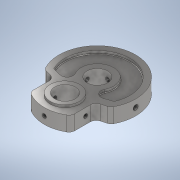
# Autodesk Inventor part: Peça10
Saved by Autodesk Inventor 2021 (Build 250183000, 183)
## iProperties
Created: 2021-07-17
Part Number: Peça10
Material: Liga de aço
Document SubType Name: Modeling
Designer: Giovanni
Density: 7.73 g/cm^3
Appearance: Semipolido
Author: Giovanni
Autodesk Inventor part; units mm, degrees
ref_plane "XZ Plane" through (0, 0, 0) normal (0, 1, 0) x (-1, 0, 0)
ref_plane "XY Plane" through (0, 0, 0) normal (0, 0, 1) x (1, 0, 0)
sketch "Esboço1" plane through (0, 0, 0) normal (0, 1, 0) x (-1, 0, 0)
  arc A0 (-55.5003, 33.8337) -> (55.5003, 33.8337) centre (0, 0) ccw
  line L0 (35, 78.734) -> (35, 47)
  line L1 (42.4118, 37.3407) -> (55.5003, 33.8337)
  line L2 (0, 0) -> (0, 90)
  arc A1 (35, 47) -> (42.4118, 37.3407) centre (45, 47) ccw
  line L3 (-35, 80.2574) -> (-35, 47)
  line L4 (-42.4118, 37.3407) -> (-55.5003, 33.8337)
  arc A2 (-42.4118, 37.3407) -> (-35, 47) centre (-45, 47) ccw
  line L5 (-35, 78.734) -> (-35, 80.2574)
  arc A3 (35, 78.734) -> (-35, 78.734) centre (0, 30) ccw
  circle A4 centre (0, 0) radius 17.5
  circle A5 centre (0, 55) radius 17.5
  point P0 (-35, 78.734)
  dimension "d6" = 65
  dimension "d7" = 90
  dimension "d8" = 35
  dimension "d9" = 105
  dimension "d10" = 10
  dimension "d11" = 47
  dimension "d12" = 10
  dimension "d13" = 35
  dimension "d14" = 105
  dimension "d15" = 60
  dimension "d16" = 35
  dimension "d17" = 55
  constraints: 12 end point, 8 point on circle, 6 centre point, 4 tangent, 4 vertical, 2 horizontal alignment, 1 coincident, 1 equal radius, 1 point on line, 1 other
  measures "d6" radius of A0
  measures "d7" distance of L2.start L2.end
  measures "d8" distance from line of L0.start L2
  measures "d9" angle of L1 L0
  measures "d10" radius of A1
  measures "d11" vertical distance of L2.start A1.centre
  measures "d12" radius of A2
  measures "d13" distance between parallel lines of L3 L2
  measures "d14" angle of L4 L3
  measures "d15" radius of A3
  measures "d16" diameter of A4
  measures "d17" distance of A5.centre L2.start
extrude "Extrusão1" add sketch "Esboço1" along normal mid plane 25
sketch "Esboço3" plane through (0, -12.5, 0) normal (0, -1, 0) x (1, 0, 0)
  arc A0 (-49.0552, 24.8713) -> (50.4541, 21.8949) centre (0, 0) ccw
  arc A1 (-23.7089, 13.9333) -> (24.4993, 12.4914) centre (0, 0) ccw
  arc A2 (-23.7089, 13.9333) -> (-34.9185, 28.6593) centre (-32.3303, 19) ccw
  line L0 (-34.9185, 28.6593) -> (-49.0552, 24.8713)
  line L1 (-42.4118, 37.3407) -> (-55.5003, 33.8337) projected
  arc A3 (36.569, 26.521) -> (24.4993, 12.4914) centre (33.4081, 17.0337) ccw
  line L2 (36.569, 26.521) -> (50.4541, 21.8949)
  dimension "d27" = 10
  dimension "d28" = 55
  dimension "d29" = 27.5
  dimension "d30" = 19
  constraints: 8 point on circle, 4 centre point, 4 end point, 4 tangent, 2 coincident, 1 equal length, 1 equal radius, 1 parallel
  measures "d27" radius of A2
  measures "d28" radius of A0
  measures "d29" radius of A1
  measures "d30" vertical distance of point (0, 0) A2.centre
extrude "Extrusão2" cut sketch "Esboço3" against normal blind 5
mirror "Espelhamento1" about plane through (0, 0, 0) normal (0, 1, 0) of "Extrusão2"
sketch "Esboço5" plane through (0, -12.5, 0) normal (0, -1, 0) x (1, 0, 0)
  circle A0 centre (0, 0) radius 23.5
  circle A1 centre (0, 0) radius 17.5 projected
  dimension "d34" = 47
  constraints: 1 centre point, 1 coincident
  measures "d34" diameter of A0
extrude "Extrusão3" add sketch "Esboço5" along normal blind 5
sketch "Esboço6" plane through (0, 12.5, 0) normal (0, 1, 0) x (1, 0, 0)
  circle A0 centre (0, -55) radius 17.5 projected
  circle A1 centre (0, -55) radius 25
  point P0 (0, 0)
  dimension "d37" = 50
  constraints: 1 centre point, 1 coincident
  measures "d37" diameter of A1
extrude "Extrusão4" add sketch "Esboço6" along normal blind 4
sketch "Esboço7" plane through (35, -12.5, 47) normal (1, 0, 0) x (0, 0, -1)
  point P0 (47, 12.5)
  point P1 (-8, 12.5)
  dimension "d40" = 55
  constraints: 1 horizontal alignment
  measures "d40" distance of point (-8, 12.5) point (47, 12.5)
hole "Furo1" at (35, 0, 55) direction (-1, 0, 0) diameter 6.917 depth 35 tip angle 118 thread size "M8x1" class "6H" standard "ANSI Metric M Profile"
pattern_circular "Padrão circular1" count 3 over 180 about axis through (0, 0, 55) along (0, -1, 0) of "Furo1"
ref_plane "Plano de trabalho1" through (65, 0, 0) normal (1, 0, 0) x (0, 1, 0)
sketch "Esboço8" plane through (65, 0, 0) normal (1, 0, 0) x (0, 1, 0)
  point P0 (0, 0)
  point P1 (0, 0)
  constraints: 1 coincident
hole "Furo2" at (65, 0, 0) direction (-1, 0, 0) diameter 8.5 depth 30
sketch "Esboço9" plane through (35, 0, 0) normal (1, 0, 0) x (0, 0, -1)
  circle A0 centre (0, 0) radius 4.25 projected
  constraints: 1 coincident
hole "Furo3" at (35, 0, 0) direction (-1, 0, 0) diameter 6.917 depth 35 thread size "M8x1" class "6H" standard "ANSI Metric M Profile"
pattern_circular "Padrão circular2" count 3 over 180 about axis through (0, 0, 0) along (0, 1, 0) of "Furo2", "Furo3"
fillet "Arredondamento1" radius 1 12 edges at (-0.8222, -7.5, -27.4877) (25.8274, -7.5, 23.5554) (43.5115, -7.5, 24.208) (-41.9869, -7.5, 26.7653) (-24.3734, -7.5, 25.057) (-1.6444, -7.5, -54.9754) (25.8274, 7.5, 23.5554) (-0.8222, 7.5, -27.4877) (-24.3734, 7.5, 25.057) (-41.9869, 7.5, 26.7653) (43.5115, 7.5, 24.208) (-1.6444, 7.5, -54.9754)
fillet "Arredondamento2" radius 10 4 edges at (-55.5003, 0, 33.8337) (-35, 0, 78.734) (55.5003, 0, 33.8337) (35, 0, 78.734)
